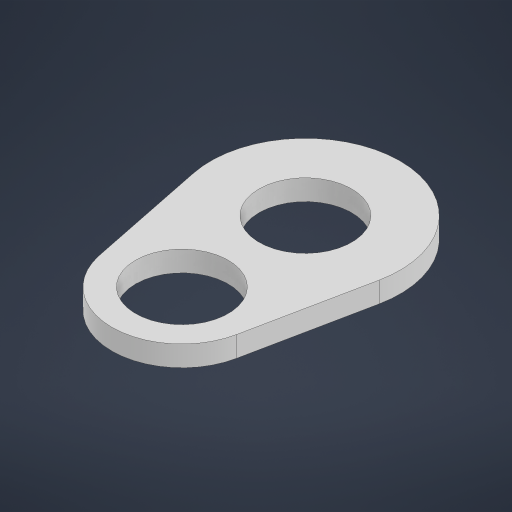
# Autodesk Inventor part: DTraining2_001_E1Base
Saved by Autodesk Inventor 2024.4 (Build 284460000, 460)
## iProperties
Created: 2026-06-11
Part Number: DTraining2_001_E1Base
Material: Generic
Document SubType Name: Modeling
Designer: hs4ho
Density: 1 g/cm^3
Appearance: Default
Author: hs4ho
Autodesk Inventor part; units mm, degrees
ref_plane "YZ Plane" through (0, 0, 0) normal (1, 0, 0) x (0, 1, 0)
ref_plane "XZ Plane" through (0, 0, 0) normal (0, 1, 0) x (-1, 0, 0)
ref_plane "XY Plane" through (0, 0, 0) normal (0, 0, 1) x (1, 0, 0)
sketch "Sketch1" plane through (0, 0, 0) normal (0, 1, 0) x (-1, 0, 0)
  circle A0 centre (0, 0) radius 15.24 construction
  circle A1 centre (0, -38.1) radius 22.86 construction
  circle A2 centre (0, 0) radius 14.2875
  circle A3 centre (0, -38.1) radius 14.2875
  line L0 (-14.9321, 3.048) -> (-22.3981, -33.528) construction
  line L1 (14.9321, 3.048) -> (22.3981, -33.528) construction
  arc A4 (-22.3981, -33.528) -> (22.3981, -33.528) centre (0, -38.1) ccw construction
  arc A5 (14.9321, 3.048) -> (-14.9321, 3.048) centre (0, 0) ccw construction
  line L2 (28.6198, -32.258) -> (21.1538, 4.318)
  arc A6 (21.1538, 4.318) -> (-21.1538, 4.318) centre (0, 0) ccw
  line L3 (-21.1538, 4.318) -> (-28.6198, -32.258)
  arc A7 (-28.6198, -32.258) -> (28.6198, -32.258) centre (0, -38.1) ccw
  dimension "d0" = 30.48
  dimension "d1" = 45.72
  dimension "d2" = 28.575
  dimension "d3" = 28.575
  dimension "d4" = 6.35
  constraints: 12 point on circle, 8 centre point, 8 end point, 8 tangent, 3 coincident, 1 equal length, 1 vertical alignment, 3 other
  measures "d0" diameter of A0
  measures "d1" diameter of A1
  measures "d2" diameter of A2
  measures "d3" diameter of A3
  measures "d4" distance between parallel lines of L1 L2
extrude "Extrusion1" add sketch "Sketch1" along normal blind 6.35
body "Solid1"
